Autodesk Inventor part; units mm, degrees
(part 5 of 8)
sketch "Skizze5" plane through (0, 0, 0) normal (0, 0, -1) x (-1, 0, 0)
  line L0 (4.6, 18.85) -> (4.6, 19.5)
  arc A0 (3.9, 18.15) -> (4.6, 18.85) centre (3.9, 18.85) ccw
  line L1 (-3.9, 18.15) -> (3.9, 18.15)
  arc A1 (-4.6, 18.85) -> (-3.9, 18.15) centre (-3.9, 18.85) ccw
  line L2 (-4.6, 19.5) -> (-4.6, 18.85)
  line L3 (-12.9, 19.5) -> (-4.6, 19.5)
  line L4 (-12.9, 14) -> (-12.9, 19.5)
  arc A2 (-14.1, 12.8) -> (-12.9, 14) centre (-14.1, 14) ccw
  line L5 (-15.5, 12.8) -> (-14.1, 12.8)
  line L6 (-15.5, -17) -> (-15.5, 12.8)
  line L7 (-13, -19.5) -> (-15.5, -17)
  line L8 (13, -19.5) -> (-13, -19.5)
  line L9 (15.5, -17) -> (13, -19.5)
  line L10 (15.5, 19.5) -> (15.5, -17)
  line L11 (4.6, 19.5) -> (15.5, 19.5)
  circle A3 centre (13.97, 2.98) radius 0.75
  circle A4 centre (13.97, 8.06) radius 0.75
  circle A5 centre (13.97, -4.64) radius 0.75
  circle A6 centre (-13.97, 8.06) radius 0.75
  circle A7 centre (-12.2, 14.85) radius 0.65
  circle A8 centre (-13.97, 0.44) radius 0.75
  circle A9 centre (-13.97, 5.52) radius 0.75
  circle A10 centre (-13.97, -2.1) radius 0.75
  line L12 (14.72, 9.85) -> (14.72, 11.35)
  line L13 (13.22, 9.85) -> (14.72, 9.85)
  line L14 (13.22, 11.35) -> (13.22, 9.85)
  line L15 (14.72, 11.35) -> (13.22, 11.35)
  circle A11 centre (13.97, -9.72) radius 0.75
  circle A12 centre (-13.97, -12.26) radius 0.75
  circle A13 centre (11.43, 8.06) radius 0.75
  circle A14 centre (-11.43, 8.06) radius 0.75
  line L16 (10.13, 5.52) -> (10.13, -12.26)
  arc A15 (12.73, 5.52) -> (10.13, 5.52) centre (11.43, 5.52) ccw
  line L17 (12.73, -12.26) -> (12.73, 5.52)
  arc A16 (10.13, -12.26) -> (12.73, -12.26) centre (11.43, -12.26) ccw
  spline S0 degree 3 poles (-6.6597, 8.2783) (-6.6601, 8.2679) (-6.6608, 8.2466) (-6.6655, 8.2142) (-6.6737, 8.1812) (-6.6829, 8.1533) (-6.6918, 8.1302) (-6.7001, 8.112) (-6.7094, 8.0929) (-6.7203, 8.0729) (-6.7319, 8.052) (-6.7451, 8.0303) (-6.7594, 8.0077) (-6.7697, 7.9925) (-6.7749, 7.9847) knots 0 0 0 0 0.09832 0.199417 0.305603 0.416162 0.474582 0.537006 0.603857 0.67409 0.749417 0.828253 0.912054 1 1 1 1
  line L18 (-6.7749, 7.9847) -> (-7.0828, 7.5344)
  line L19 (-7.0828, 7.5344) -> (-7.1545, 7.5842)
  line L20 (-7.1545, 7.5842) -> (-6.8765, 7.9907)
  spline S1 degree 3 poles (-6.8765, 7.9907) (-6.8942, 7.9885) (-6.9292, 7.9842) (-6.9643, 7.9835) (-6.9817, 7.9831) knots 0 0 0 0 0.507858 1 1 1 1
  spline S2 degree 3 poles (-6.9817, 7.9831) (-6.9922, 7.9833) (-7.0128, 7.9839) (-7.0431, 7.9881) (-7.0722, 7.9945) (-7.1, 8.0041) (-7.1267, 8.0161) (-7.1522, 8.0309) (-7.1764, 8.0483) (-7.1991, 8.0683) (-7.2198, 8.0902) (-7.2382, 8.1134) (-7.2535, 8.1381) (-7.2662, 8.1639) (-7.2758, 8.1911) (-7.2829, 8.2194) (-7.2872, 8.249) (-7.2877, 8.2691) (-7.2879, 8.2794) knots 0 0 0 0 0.066295 0.130131 0.192862 0.25436 0.31591 0.377338 0.440205 0.504175 0.568034 0.630228 0.690861 0.751422 0.811466 0.87275 0.935391 1 1 1 1
  spline S3 degree 3 poles (-7.2879, 8.2794) (-7.2875, 8.2933) (-7.2865, 8.3208) (-7.2787, 8.3609) (-7.2658, 8.3989) (-7.2478, 8.4345) (-7.2252, 8.4674) (-7.198, 8.497) (-7.1665, 8.5229) (-7.1312, 8.5452) (-7.0931, 8.5631) (-7.0532, 8.5763) (-7.0118, 8.5841) (-6.9838, 8.5851) (-6.9696, 8.5856) knots 0 0 0 0 0.085249 0.167327 0.248175 0.328829 0.409908 0.490584 0.572993 0.658265 0.744222 0.82906 0.913938 1 1 1 1
  spline S4 degree 3 poles (-6.9696, 8.5856) (-6.9558, 8.5851) (-6.9284, 8.5841) (-6.8882, 8.5765) (-6.8496, 8.5638) (-6.813, 8.5461) (-6.779, 8.524) (-6.7485, 8.4977) (-6.7221, 8.4672) (-6.6999, 8.4331) (-6.6821, 8.3965) (-6.6692, 8.3582) (-6.6612, 8.3187) (-6.6602, 8.2919) (-6.6597, 8.2783) knots 0 0 0 0 0.085532 0.169003 0.251943 0.335682 0.419409 0.501265 0.583703 0.668 0.751919 0.834598 0.916526 1 1 1 1
  line L21 (-3.0444, 5.02) -> (-3.0572, 5.02)
  line L22 (-3.0572, 5.02) -> (-3.4803, 6.02)
  line L23 (-3.4803, 6.02) -> (-3.3841, 6.02)
  line L24 (-3.3841, 6.02) -> (-3.0508, 5.2319)
  line L25 (-3.0508, 5.2319) -> (-2.7174, 6.02)
  line L26 (-2.7174, 6.02) -> (-2.6213, 6.02)
  line L27 (-2.6213, 6.02) -> (-3.0444, 5.02)
  spline S5 degree 3 poles (-3.7238, 5.7862) (-3.724, 5.7914) (-3.7242, 5.8018) (-3.7272, 5.817) (-3.7316, 5.8317) (-3.7378, 5.8459) (-3.746, 5.8595) (-3.7558, 5.8725) (-3.7675, 5.885) (-3.7809, 5.8966) (-3.7953, 5.9077) (-3.8111, 5.9171) (-3.8278, 5.9251) (-3.8454, 5.9318) (-3.864, 5.9368) (-3.8835, 5.9404) (-3.9039, 5.9426) (-3.9179, 5.9429) (-3.925, 5.9431) knots 0 0 0 0 0.055275 0.109966 0.163247 0.218076 0.273301 0.330909 0.390995 0.454176 0.518862 0.583311 0.648517 0.715031 0.782502 0.852323 0.924928 1 1 1 1
  spline S6 degree 3 poles (-3.925, 5.9431) (-3.9364, 5.9427) (-3.9586, 5.9419) (-3.9907, 5.9351) (-4.0205, 5.9243) (-4.0432, 5.9113) (-4.0601, 5.8985) (-4.0721, 5.8873) (-4.0839, 5.8749) (-4.0947, 5.8605) (-4.1056, 5.8451) (-4.1156, 5.8278) (-4.1253, 5.8092) (-4.1311, 5.796) (-4.1341, 5.7892) knots 0 0 0 0 0.122712 0.239685 0.351816 0.463766 0.520818 0.579448 0.640604 0.705298 0.773634 0.844669 0.920057 1 1 1 1
  line L28 (-4.1341, 5.7892) -> (-4.2238, 5.7892)
  spline S7 degree 3 poles (-4.2238, 5.7892) (-4.2214, 5.7993) (-4.2167, 5.819) (-4.2067, 5.8471) (-4.1959, 5.8737) (-4.183, 5.8983) (-4.1688, 5.9214) (-4.1526, 5.9424) (-4.1351, 5.962) (-4.1157, 5.9793) (-4.0954, 5.995) (-4.0739, 6.0084) (-4.0515, 6.0199) (-4.0282, 6.0294) (-4.0039, 6.0366) (-3.9788, 6.0418) (-3.9528, 6.0451) (-3.9351, 6.0455) (-3.9262, 6.0456) knots 0 0 0 0 0.072625 0.141977 0.208985 0.273957 0.336889 0.398745 0.460116 0.520825 0.580994 0.640152 0.698622 0.757271 0.816427 0.876254 0.937165 1 1 1 1
  spline S8 degree 3 poles (-3.9262, 6.0456) (-3.9131, 6.0452) (-3.8873, 6.0445) (-3.8494, 6.0373) (-3.8128, 6.0261) (-3.778, 6.0105) (-3.7456, 5.9913) (-3.7168, 5.9685) (-3.692, 5.9424) (-3.6712, 5.9136) (-3.6549, 5.8829) (-3.6428, 5.8512) (-3.6355, 5.8187) (-3.6346, 5.7968) (-3.6341, 5.7858) knots 0 0 0 0 0.090254 0.17854 0.266093 0.354631 0.441886 0.525747 0.608114 0.690197 0.770821 0.848326 0.924012 1 1 1 1
  spline S9 degree 3 poles (-3.6341, 5.7858) (-3.6344, 5.7753) (-3.6351, 5.7546) (-3.6406, 5.7244) (-3.6499, 5.6959) (-3.6628, 5.669) (-3.6795, 5.644) (-3.6996, 5.6206) (-3.7235, 5.5989) (-3.7416, 5.5865) (-3.7509, 5.5801) knots 0 0 0 0 0.128068 0.250608 0.37063 0.490072 0.610375 0.734313 0.863217 1 1 1 1
  spline S10 degree 3 poles (-3.7509, 5.5801) (-3.7403, 5.575) (-3.7192, 5.5648) (-3.6904, 5.5448) (-3.6644, 5.5218) (-3.6498, 5.5038) (-3.6425, 5.4948) knots 0 0 0 0 0.25388 0.503009 0.750291 1 1 1 1
  spline S11 degree 3 poles (-3.6425, 5.4948) (-3.6377, 5.4882) (-3.6282, 5.4751) (-3.6164, 5.4541) (-3.6057, 5.4329) (-3.5974, 5.4108) (-3.5909, 5.3882) (-3.5863, 5.365) (-3.5834, 5.3413) (-3.583, 5.3252) (-3.5828, 5.3171) knots 0 0 0 0 0.128136 0.254173 0.378112 0.501712 0.623986 0.747096 0.872875 1 1 1 1
  spline S12 degree 3 poles (-3.5828, 5.3171) (-3.5833, 5.3031) (-3.5844, 5.2751) (-3.5935, 5.2339) (-3.6077, 5.1935) (-3.6278, 5.1549) (-3.6523, 5.1188) (-3.6815, 5.0865) (-3.715, 5.0587) (-3.7524, 5.0355) (-3.7929, 5.017) (-3.8362, 5.0041) (-3.8817, 4.9957) (-3.9129, 4.9948) (-3.9288, 4.9944) knots 0 0 0 0 0.079648 0.158922 0.239619 0.322609 0.406035 0.487602 0.569685 0.653036 0.737436 0.822478 0.909748 1 1 1 1
  spline S13 degree 3 poles (-3.9288, 4.9944) (-3.9395, 4.9946) (-3.9605, 4.9951) (-3.9914, 4.9984) (-4.0209, 5.0045) (-4.0491, 5.0127) (-4.0759, 5.0231) (-4.1013, 5.0361) (-4.1254, 5.0513) (-4.1481, 5.069) (-4.1692, 5.0888) (-4.1883, 5.111) (-4.2056, 5.1353) (-4.2207, 5.1619) (-4.2343, 5.1905) (-4.2455, 5.2214) (-4.2554, 5.2544) (-4.26, 5.2774) (-4.2623, 5.2892) knots 0 0 0 0 0.065541 0.128963 0.190377 0.250092 0.308548 0.366398 0.424542 0.48317 0.542243 0.601739 0.662506 0.724856 0.789128 0.856346 0.926295 1 1 1 1
  line L29 (-4.2623, 5.2892) -> (-4.1726, 5.2892)
  spline S14 degree 3 poles (-4.1726, 5.2892) (-4.1702, 5.2815) (-4.1657, 5.2666) (-4.1579, 5.245) (-4.1491, 5.2252) (-4.1397, 5.2071) (-4.1297, 5.1905) (-4.1186, 5.1758) (-4.1071, 5.1623) (-4.0985, 5.1547) (-4.0942, 5.151) knots 0 0 0 0 0.14977 0.291316 0.425966 0.55216 0.671527 0.786122 0.895325 1 1 1 1
  spline S15 degree 3 poles (-4.0942, 5.151) (-4.0886, 5.1467) (-4.0775, 5.1381) (-4.0592, 5.1271) (-4.0401, 5.1175) (-4.0196, 5.1103) (-3.9981, 5.1041) (-3.9754, 5.1001) (-3.9517, 5.0973) (-3.9355, 5.097) (-3.9272, 5.0969) knots 0 0 0 0 0.118271 0.236178 0.355663 0.475904 0.600127 0.728608 0.861313 1 1 1 1
  spline S16 degree 3 poles (-3.9272, 5.0969) (-3.9178, 5.0971) (-3.8995, 5.0974) (-3.8728, 5.1006) (-3.8474, 5.1052) (-3.8236, 5.1123) (-3.801, 5.1211) (-3.7801, 5.1322) (-3.7604, 5.1451) (-3.7423, 5.1599) (-3.7261, 5.176) (-3.7117, 5.1928) (-3.6995, 5.2104) (-3.6897, 5.2287) (-3.682, 5.2476) (-3.6767, 5.2674) (-3.673, 5.2877) (-3.6727, 5.3015) (-3.6726, 5.3085) knots 0 0 0 0 0.076072 0.148752 0.218403 0.28576 0.350598 0.414964 0.478069 0.541761 0.60435 0.664075 0.721464 0.777587 0.832644 0.887844 0.94346 1 1 1 1
  spline S17 degree 3 poles (-3.6726, 5.3085) (-3.673, 5.3178) (-3.6739, 5.3364) (-3.6805, 5.3637) (-3.6915, 5.3901) (-3.7068, 5.415) (-3.7255, 5.438) (-3.7473, 5.4586) (-3.7725, 5.4756) (-3.7956, 5.4874) (-3.8161, 5.4954) (-3.8337, 5.5007) (-3.8533, 5.5052) (-3.8748, 5.5094) (-3.8983, 5.513) (-3.9239, 5.516) (-3.9514, 5.5184) (-3.9704, 5.5195) (-3.9803, 5.52) knots 0 0 0 0 0.066909 0.133485 0.201035 0.271234 0.34288 0.413836 0.485977 0.56023 0.599884 0.644055 0.691892 0.744688 0.801492 0.862858 0.929328 1 1 1 1
  line L30 (-3.9803, 5.52) -> (-3.9803, 5.6226)
  spline S18 degree 3 poles (-3.9803, 5.6226) (-3.9679, 5.6228) (-3.9437, 5.6232) (-3.9083, 5.6282) (-3.8744, 5.635) (-3.8429, 5.6456) (-3.8141, 5.6578) (-3.7891, 5.6721) (-3.7684, 5.6879) (-3.7518, 5.7056) (-3.7394, 5.7245) (-3.7303, 5.7443) (-3.7249, 5.765) (-3.7242, 5.7791) (-3.7238, 5.7862) knots 0 0 0 0 0.110166 0.215787 0.318027 0.417574 0.51165 0.596162 0.672935 0.74367 0.810677 0.874059 0.936696 1 1 1 1
  spline S19 degree 3 poles (-4.4738, 5.0072) (-4.4794, 5.0075) (-4.4903, 5.0081) (-4.506, 5.013) (-4.5204, 5.0206) (-4.5332, 5.0313) (-4.5436, 5.0441) (-4.5515, 5.0585) (-4.5562, 5.0741) (-4.5569, 5.085) (-4.5572, 5.0905) knots 0 0 0 0 0.127757 0.249414 0.372796 0.500111 0.62861 0.750643 0.873768 1 1 1 1
  spline S20 degree 3 poles (-4.5572, 5.0905) (-4.5569, 5.0962) (-4.5563, 5.1072) (-4.5515, 5.1229) (-4.5437, 5.1373) (-4.5331, 5.15) (-4.5204, 5.1606) (-4.506, 5.1683) (-4.4903, 5.1729) (-4.4794, 5.1735) (-4.4738, 5.1738) knots 0 0 0 0 0.129097 0.252046 0.373905 0.501038 0.628171 0.751376 0.872426 1 1 1 1
  spline S21 degree 3 poles (-4.4738, 5.1738) (-4.4683, 5.1735) (-4.4574, 5.1729) (-4.4416, 5.1684) (-4.4273, 5.1605) (-4.4146, 5.15) (-4.4041, 5.1372) (-4.3959, 5.123) (-4.3915, 5.1071) (-4.3908, 5.0961) (-4.3905, 5.0905) knots 0 0 0 0 0.127519 0.249986 0.371792 0.49887 0.625948 0.748492 0.870959 1 1 1 1
  spline S22 degree 3 poles (-4.3905, 5.0905) (-4.3909, 5.085) (-4.3915, 5.0742) (-4.3959, 5.0584) (-4.4041, 5.0442) (-4.4145, 5.0313) (-4.4273, 5.0207) (-4.4416, 5.0129) (-4.4573, 5.0081) (-4.4683, 5.0075) (-4.4738, 5.0072) knots 0 0 0 0 0.126178 0.248821 0.37154 0.499984 0.627244 0.749226 0.872298 1 1 1 1
  spline S23 degree 3 poles (-4.8649, 5.7862) (-4.865, 5.7914) (-4.8652, 5.8018) (-4.8682, 5.817) (-4.8727, 5.8317) (-4.8788, 5.8459) (-4.887, 5.8595) (-4.8968, 5.8725) (-4.9085, 5.885) (-4.922, 5.8966) (-4.9364, 5.9077) (-4.9521, 5.9171) (-4.9688, 5.9251) (-4.9865, 5.9318) (-5.0051, 5.9368) (-5.0246, 5.9404) (-5.045, 5.9426) (-5.0589, 5.9429) (-5.066, 5.9431) knots 0 0 0 0 0.055275 0.109966 0.163247 0.218076 0.273301 0.330909 0.390995 0.454176 0.518862 0.583311 0.648517 0.715031 0.782502 0.852323 0.924928 1 1 1 1
  spline S24 degree 3 poles (-5.066, 5.9431) (-5.0774, 5.9427) (-5.0996, 5.9419) (-5.1317, 5.9351) (-5.1615, 5.9243) (-5.1843, 5.9113) (-5.2011, 5.8985) (-5.2131, 5.8873) (-5.2249, 5.8749) (-5.2357, 5.8605) (-5.2467, 5.8451) (-5.2566, 5.8278) (-5.2663, 5.8092) (-5.2721, 5.796) (-5.2751, 5.7892) knots 0 0 0 0 0.122712 0.239685 0.351816 0.463766 0.520818 0.579448 0.640604 0.705298 0.773634 0.844669 0.920057 1 1 1 1
  line L31 (-5.2751, 5.7892) -> (-5.3649, 5.7892)
  spline S25 degree 3 poles (-5.3649, 5.7892) (-5.3624, 5.7993) (-5.3577, 5.819) (-5.3478, 5.8471) (-5.337, 5.8737) (-5.324, 5.8983) (-5.3099, 5.9214) (-5.2937, 5.9424) (-5.2761, 5.962) (-5.2568, 5.9793) (-5.2364, 5.995) (-5.2149, 6.0084) (-5.1925, 6.0199) (-5.1692, 6.0294) (-5.1449, 6.0366) (-5.1198, 6.0418) (-5.0938, 6.0451) (-5.0762, 6.0455) (-5.0672, 6.0456) knots 0 0 0 0 0.072625 0.141977 0.208985 0.273957 0.336889 0.398745 0.460116 0.520825 0.580994 0.640152 0.698622 0.757271 0.816427 0.876254 0.937165 1 1 1 1
  spline S26 degree 3 poles (-5.0672, 6.0456) (-5.0541, 6.0452) (-5.0283, 6.0445) (-4.9904, 6.0373) (-4.9538, 6.0261) (-4.919, 6.0105) (-4.8866, 5.9913) (-4.8579, 5.9685) (-4.833, 5.9424) (-4.8122, 5.9136) (-4.7959, 5.8829) (-4.7839, 5.8512) (-4.7766, 5.8187) (-4.7756, 5.7968) (-4.7751, 5.7858) knots 0 0 0 0 0.090254 0.17854 0.266093 0.354631 0.441886 0.525747 0.608114 0.690197 0.770821 0.848326 0.924012 1 1 1 1
  spline S27 degree 3 poles (-4.7751, 5.7858) (-4.7755, 5.7753) (-4.7761, 5.7546) (-4.7816, 5.7244) (-4.7909, 5.6959) (-4.8038, 5.669) (-4.8205, 5.644) (-4.8407, 5.6206) (-4.8645, 5.5989) (-4.8826, 5.5865) (-4.8919, 5.5801) knots 0 0 0 0 0.128068 0.250608 0.37063 0.490072 0.610375 0.734313 0.863217 1 1 1 1
  spline S28 degree 3 poles (-4.8919, 5.5801) (-4.8813, 5.575) (-4.8602, 5.5648) (-4.8315, 5.5448) (-4.8054, 5.5218) (-4.7908, 5.5038) (-4.7835, 5.4948) knots 0 0 0 0 0.25388 0.503009 0.750291 1 1 1 1
  spline S29 degree 3 poles (-4.7835, 5.4948) (-4.7787, 5.4882) (-4.7692, 5.4751) (-4.7574, 5.4541) (-4.7467, 5.4329) (-4.7384, 5.4108) (-4.7319, 5.3882) (-4.7273, 5.365) (-4.7245, 5.3413) (-4.7241, 5.3252) (-4.7238, 5.3171) knots 0 0 0 0 0.128136 0.254173 0.378112 0.501712 0.623986 0.747096 0.872875 1 1 1 1
  spline S30 degree 3 poles (-4.7238, 5.3171) (-4.7244, 5.3031) (-4.7254, 5.2751) (-4.7345, 5.2339) (-4.7487, 5.1935) (-4.7688, 5.1549) (-4.7934, 5.1188) (-4.8226, 5.0865) (-4.8561, 5.0587) (-4.8934, 5.0355) (-4.9339, 5.017) (-4.9772, 5.0041) (-5.0227, 4.9957) (-5.0539, 4.9948) (-5.0698, 4.9944) knots 0 0 0 0 0.079648 0.158922 0.239619 0.322609 0.406035 0.487602 0.569685 0.653036 0.737436 0.822478 0.909748 1 1 1 1
  spline S31 degree 3 poles (-5.0698, 4.9944) (-5.0805, 4.9946) (-5.1015, 4.9951) (-5.1325, 4.9984) (-5.162, 5.0045) (-5.1901, 5.0127) (-5.2169, 5.0231) (-5.2423, 5.0361) (-5.2665, 5.0513) (-5.2891, 5.069) (-5.3102, 5.0888) (-5.3293, 5.111) (-5.3466, 5.1353) (-5.3617, 5.1619) (-5.3754, 5.1905) (-5.3865, 5.2214) (-5.3964, 5.2544) (-5.401, 5.2774) (-5.4033, 5.2892) knots 0 0 0 0 0.065541 0.128963 0.190377 0.250092 0.308548 0.366398 0.424542 0.48317 0.542243 0.601739 0.662506 0.724856 0.789128 0.856346 0.926295 1 1 1 1
  line L32 (-5.4033, 5.2892) -> (-5.3136, 5.2892)
  spline S32 degree 3 poles (-5.3136, 5.2892) (-5.3113, 5.2815) (-5.3067, 5.2666) (-5.299, 5.245) (-5.2901, 5.2252) (-5.2807, 5.2071) (-5.2707, 5.1905) (-5.2596, 5.1758) (-5.2481, 5.1623) (-5.2395, 5.1547) (-5.2353, 5.151) knots 0 0 0 0 0.14977 0.291316 0.425966 0.55216 0.671527 0.786122 0.895325 1 1 1 1
  spline S33 degree 3 poles (-5.2353, 5.151) (-5.2297, 5.1467) (-5.2185, 5.1381) (-5.2003, 5.1271) (-5.1811, 5.1175) (-5.1606, 5.1103) (-5.1392, 5.1041) (-5.1165, 5.1001) (-5.0927, 5.0973) (-5.0765, 5.097) (-5.0682, 5.0969) knots 0 0 0 0 0.118271 0.236178 0.355663 0.475904 0.600127 0.728608 0.861313 1 1 1 1
  spline S34 degree 3 poles (-5.0682, 5.0969) (-5.0588, 5.0971) (-5.0405, 5.0974) (-5.0138, 5.1006) (-4.9884, 5.1052) (-4.9646, 5.1123) (-4.9421, 5.1211) (-4.9211, 5.1322) (-4.9014, 5.1451) (-4.8833, 5.1599) (-4.8671, 5.176) (-4.8528, 5.1928) (-4.8406, 5.2104) (-4.8307, 5.2287) (-4.823, 5.2476) (-4.8177, 5.2674) (-4.814, 5.2877) (-4.8137, 5.3015) (-4.8136, 5.3085) knots 0 0 0 0 0.076072 0.148752 0.218403 0.28576 0.350598 0.414964 0.478069 0.541761 0.60435 0.664075 0.721464 0.777587 0.832644 0.887844 0.94346 1 1 1 1
  spline S35 degree 3 poles (-4.8136, 5.3085) (-4.814, 5.3178) (-4.8149, 5.3364) (-4.8216, 5.3637) (-4.8325, 5.3901) (-4.8478, 5.415) (-4.8665, 5.438) (-4.8883, 5.4586) (-4.9135, 5.4756) (-4.9366, 5.4874) (-4.9571, 5.4954) (-4.9747, 5.5007) (-4.9943, 5.5052) (-5.0158, 5.5094) (-5.0394, 5.513) (-5.0649, 5.516) (-5.0924, 5.5184) (-5.1115, 5.5195) (-5.1213, 5.52) knots 0 0 0 0 0.066909 0.133485 0.201035 0.271234 0.34288 0.413836 0.485977 0.56023 0.599884 0.644055 0.691892 0.744688 0.801492 0.862858 0.929328 1 1 1 1
  line L33 (-5.1213, 5.52) -> (-5.1213, 5.6226)
  spline S36 degree 3 poles (-5.1213, 5.6226) (-5.1089, 5.6228) (-5.0847, 5.6232) (-5.0493, 5.6282) (-5.0154, 5.635) (-4.9839, 5.6456) (-4.9551, 5.6578) (-4.9302, 5.6721) (-4.9094, 5.6879) (-4.8929, 5.7056) (-4.8804, 5.7245) (-4.8713, 5.7443) (-4.8659, 5.765) (-4.8652, 5.7791) (-4.8649, 5.7862) knots 0 0 0 0 0.110166 0.215787 0.318027 0.417574 0.51165 0.596162 0.672935 0.74367 0.810677 0.874059 0.936696 1 1 1 1
  spline S37 degree 3 poles (-3.3905, 2.9796) (-3.3907, 2.9643) (-3.3911, 2.9345) (-3.3929, 2.8909) (-3.3966, 2.8498) (-3.4013, 2.811) (-3.4077, 2.7747) (-3.4156, 2.7408) (-3.4243, 2.7091) (-3.4351, 2.6798) (-3.447, 2.6527) (-3.4598, 2.6274) (-3.4736, 2.6036) (-3.4887, 2.5816) (-3.5047, 2.5612) (-3.522, 2.5428) (-3.5402, 2.5259) (-3.5595, 2.5109) (-3.5796, 2.4977) (-3.6002, 2.4859) (-3.6215, 2.4764) (-3.6432, 2.4683) (-3.6655, 2.462) (-3.6885, 2.4577) (-3.7119, 2.4547) (-3.7277, 2.4545) (-3.7357, 2.4544) knots 0 0 0 0 0.065063 0.126773 0.185516 0.240765 0.29298 0.34225 0.388919 0.432776 0.474628 0.514775 0.553606 0.591426 0.628028 0.663804 0.698984 0.733591 0.767628 0.801208 0.834264 0.866981 0.89972 0.932702 0.966176 1 1 1 1
  spline S38 degree 3 poles (-3.7357, 2.4544) (-3.7436, 2.4545) (-3.7591, 2.4548) (-3.7821, 2.4575) (-3.8045, 2.4618) (-3.8263, 2.468) (-3.8477, 2.4755) (-3.8683, 2.4852) (-3.8883, 2.4964) (-3.9079, 2.5092) (-3.9264, 2.5239) (-3.9442, 2.5401) (-3.9606, 2.5583) (-3.976, 2.5782) (-3.9905, 2.5995) (-4.0039, 2.6226) (-4.0163, 2.6474) (-4.0276, 2.6741) (-4.0377, 2.703) (-4.0465, 2.7345) (-4.0536, 2.7688) (-4.0595, 2.8057) (-4.0644, 2.8453) (-4.0677, 2.8877) (-4.0697, 2.9328) (-4.0699, 2.9637) (-4.07, 2.9796) knots 0 0 0 0 0.033787 0.066622 0.099285 0.131361 0.163585 0.196104 0.228902 0.262158 0.295991 0.330218 0.36506 0.400951 0.43762 0.475708 0.515381 0.556414 0.599765 0.646424 0.696431 0.749782 0.806573 0.867436 0.931887 1 1 1 1
  spline S39 degree 3 poles (-4.07, 2.9796) (-4.0699, 2.9956) (-4.0697, 3.0268) (-4.0677, 3.0721) (-4.0643, 3.1147) (-4.0597, 3.1544) (-4.0541, 3.1914) (-4.0466, 3.2255) (-4.0381, 3.2568) (-4.0282, 3.2855) (-4.0171, 3.312) (-4.005, 3.3366) (-3.9914, 3.3595) (-3.9771, 3.381) (-3.9616, 3.4007) (-3.9452, 3.4189) (-3.9273, 3.4351) (-3.9087, 3.45) (-3.8889, 3.4629) (-3.8688, 3.4744) (-3.848, 3.4841) (-3.8265, 3.4918) (-3.8046, 3.4982) (-3.7821, 3.5025) (-3.7591, 3.5052) (-3.7436, 3.5055) (-3.7357, 3.5056) knots 0 0 0 0 0.068595 0.133246 0.194313 0.251279 0.304513 0.354235 0.400481 0.443411 0.484015 0.523252 0.561042 0.5979 0.633518 0.668314 0.702496 0.736685 0.770293 0.803437 0.835913 0.86846 0.900847 0.933467 0.966258 1 1 1 1
  spline S40 degree 3 poles (-3.7357, 3.5056) (-3.7277, 3.5055) (-3.7119, 3.5052) (-3.6885, 3.5026) (-3.6657, 3.4981) (-3.6435, 3.4919) (-3.6217, 3.4841) (-3.6006, 3.4744) (-3.58, 3.463) (-3.5602, 3.4497) (-3.5409, 3.4349) (-3.5228, 3.4181) (-3.5058, 3.3995) (-3.4896, 3.3794) (-3.4747, 3.3573) (-3.4605, 3.3337) (-3.4479, 3.308) (-3.4356, 3.2808) (-3.4251, 3.2513) (-3.4156, 3.2197) (-3.4079, 3.1855) (-3.4015, 3.149) (-3.3966, 3.11) (-3.393, 3.0687) (-3.3911, 3.0249) (-3.3907, 2.995) (-3.3905, 2.9796) knots 0 0 0 0 0.033788 0.067194 0.099862 0.132567 0.165151 0.197913 0.231319 0.265083 0.299255 0.334399 0.369943 0.406284 0.444064 0.482998 0.523354 0.565537 0.609613 0.656391 0.705885 0.758325 0.813832 0.872795 0.934722 1 1 1 1
  spline S41 degree 3 poles (-2.7623, 0.7062) (-2.7624, 0.7114) (-2.7627, 0.7218) (-2.7656, 0.737) (-2.7701, 0.7517) (-2.7762, 0.7659) (-2.7844, 0.7795) (-2.7943, 0.7925) (-2.806, 0.805) (-2.8194, 0.8166) (-2.8338, 0.8277) (-2.8496, 0.8371) (-2.8663, 0.8451) (-2.8839, 0.8518) (-2.9025, 0.8568) (-2.922, 0.8604) (-2.9424, 0.8626) (-2.9563, 0.8629) (-2.9634, 0.8631) knots 0 0 0 0 0.055275 0.109966 0.163247 0.218076 0.273301 0.330909 0.390995 0.454176 0.518862 0.583311 0.648517 0.715031 0.782502 0.852323 0.924928 1 1 1 1
  spline S42 degree 3 poles (-2.9634, 0.8631) (-2.9748, 0.8627) (-2.9971, 0.8619) (-3.0291, 0.8551) (-3.0589, 0.8443) (-3.0817, 0.8313) (-3.0985, 0.8185) (-3.1106, 0.8073) (-3.1224, 0.7949) (-3.1332, 0.7805) (-3.1441, 0.7651) (-3.1541, 0.7478) (-3.1637, 0.7292) (-3.1696, 0.716) (-3.1726, 0.7092) knots 0 0 0 0 0.122712 0.239685 0.351816 0.463766 0.520818 0.579448 0.640604 0.705298 0.773634 0.844669 0.920057 1 1 1 1
  line L34 (-3.1726, 0.7092) -> (-3.2623, 0.7092)
  spline S43 degree 3 poles (-3.2623, 0.7092) (-3.2599, 0.7193) (-3.2551, 0.739) (-3.2452, 0.7671) (-3.2344, 0.7937) (-3.2214, 0.8183) (-3.2073, 0.8414) (-3.1911, 0.8624) (-3.1736, 0.882) (-3.1542, 0.8993) (-3.1339, 0.915) (-3.1123, 0.9284) (-3.09, 0.9399) (-3.0667, 0.9494) (-3.0423, 0.9566) (-3.0172, 0.9618) (-2.9912, 0.9651) (-2.9736, 0.9655) (-2.9646, 0.9656) knots 0 0 0 0 0.072625 0.141977 0.208985 0.273957 0.336889 0.398745 0.460116 0.520825 0.580994 0.640152 0.698622 0.757271 0.816427 0.876254 0.937165 1 1 1 1
  spline S44 degree 3 poles (-2.9646, 0.9656) (-2.9516, 0.9652) (-2.9258, 0.9645) (-2.8878, 0.9573) (-2.8512, 0.9461) (-2.8164, 0.9305) (-2.7841, 0.9113) (-2.7553, 0.8885) (-2.7305, 0.8624) (-2.7096, 0.8336) (-2.6933, 0.8029) (-2.6813, 0.7712) (-2.674, 0.7387) (-2.673, 0.7168) (-2.6726, 0.7058) knots 0 0 0 0 0.090254 0.17854 0.266093 0.354631 0.441886 0.525747 0.608114 0.690197 0.770821 0.848326 0.924012 1 1 1 1
  spline S45 degree 3 poles (-2.6726, 0.7058) (-2.6729, 0.6953) (-2.6735, 0.6746) (-2.6791, 0.6444) (-2.6884, 0.6159) (-2.7012, 0.589) (-2.7179, 0.564) (-2.7381, 0.5406) (-2.762, 0.5189) (-2.78, 0.5065) (-2.7894, 0.5001) knots 0 0 0 0 0.128068 0.250608 0.37063 0.490072 0.610375 0.734313 0.863217 1 1 1 1
  spline S46 degree 3 poles (-2.7894, 0.5001) (-2.7787, 0.495) (-2.7576, 0.4848) (-2.7289, 0.4648) (-2.7028, 0.4418) (-2.6883, 0.4238) (-2.681, 0.4148) knots 0 0 0 0 0.25388 0.503009 0.750291 1 1 1 1
  spline S47 degree 3 poles (-2.681, 0.4148) (-2.6762, 0.4082) (-2.6666, 0.3951) (-2.6548, 0.3741) (-2.6442, 0.3529) (-2.6358, 0.3308) (-2.6294, 0.3082) (-2.6248, 0.285) (-2.6219, 0.2613) (-2.6215, 0.2452) (-2.6213, 0.2371) knots 0 0 0 0 0.128136 0.254173 0.378112 0.501712 0.623986 0.747096 0.872875 1 1 1 1
  spline S48 degree 3 poles (-2.6213, 0.2371) (-2.6218, 0.2231) (-2.6228, 0.1951) (-2.632, 0.1539) (-2.6461, 0.1135) (-2.6663, 0.0749) (-2.6908, 0.0388) (-2.72, 0.0065) (-2.7535, -0.0213) (-2.7909, -0.0445) (-2.8314, -0.063) (-2.8747, -0.0759) (-2.9202, -0.0843) (-2.9514, -0.0852) (-2.9672, -0.0856) knots 0 0 0 0 0.079648 0.158922 0.239619 0.322609 0.406035 0.487602 0.569685 0.653036 0.737436 0.822478 0.909748 1 1 1 1
  spline S49 degree 3 poles (-2.9672, -0.0856) (-2.9779, -0.0854) (-2.999, -0.0849) (-3.0299, -0.0816) (-3.0594, -0.0755) (-3.0876, -0.0673) (-3.1144, -0.0569) (-3.1398, -0.0439) (-3.1639, -0.0287) (-3.1865, -0.011) (-3.2076, 0.0088) (-3.2267, 0.031) (-3.2441, 0.0553) (-3.2592, 0.0819) (-3.2728, 0.1105) (-3.284, 0.1414) (-3.2938, 0.1744) (-3.2984, 0.1974) (-3.3008, 0.2092) knots 0 0 0 0 0.065541 0.128963 0.190377 0.250092 0.308548 0.366398 0.424542 0.48317 0.542243 0.601739 0.662506 0.724856 0.789128 0.856346 0.926295 1 1 1 1
  line L35 (-3.3008, 0.2092) -> (-3.211, 0.2092)
  spline S50 degree 3 poles (-3.211, 0.2092) (-3.2087, 0.2015) (-3.2041, 0.1866) (-3.1964, 0.165) (-3.1876, 0.1452) (-3.1781, 0.1271) (-3.1682, 0.1105) (-3.1571, 0.0958) (-3.1456, 0.0823) (-3.1369, 0.0747) (-3.1327, 0.071) knots 0 0 0 0 0.14977 0.291316 0.425966 0.55216 0.671527 0.786122 0.895325 1 1 1 1
  spline S51 degree 3 poles (-3.1327, 0.071) (-3.1271, 0.0667) (-3.1159, 0.0581) (-3.0977, 0.0471) (-3.0785, 0.0375) (-3.058, 0.0303) (-3.0366, 0.0241) (-3.0139, 0.0201) (-2.9901, 0.0173) (-2.9739, 0.017) (-2.9656, 0.0169) knots 0 0 0 0 0.118271 0.236178 0.355663 0.475904 0.600127 0.728608 0.861313 1 1 1 1
  spline S52 degree 3 poles (-2.9656, 0.0169) (-2.9563, 0.0171) (-2.938, 0.0174) (-2.9113, 0.0206) (-2.8859, 0.0252) (-2.8621, 0.0323) (-2.8395, 0.0411) (-2.8185, 0.0522) (-2.7989, 0.0651) (-2.7808, 0.0799) (-2.7645, 0.096) (-2.7502, 0.1128) (-2.738, 0.1304) (-2.7282, 0.1487) (-2.7204, 0.1676) (-2.7151, 0.1874) (-2.7115, 0.2077) (-2.7112, 0.2215) (-2.711, 0.2285) knots 0 0 0 0 0.076072 0.148752 0.218403 0.28576 0.350598 0.414964 0.478069 0.541761 0.60435 0.664075 0.721464 0.777587 0.832644 0.887844 0.94346 1 1 1 1
  spline S53 degree 3 poles (-2.711, 0.2285) (-2.7115, 0.2378) (-2.7123, 0.2564) (-2.719, 0.2837) (-2.7299, 0.3101) (-2.7453, 0.335) (-2.764, 0.358) (-2.7858, 0.3786) (-2.8109, 0.3956) (-2.8341, 0.4074) (-2.8546, 0.4154) (-2.8721, 0.4207) (-2.8918, 0.4252) (-2.9133, 0.4294) (-2.9368, 0.433) (-2.9623, 0.436) (-2.9898, 0.4384) (-3.0089, 0.4395) (-3.0187, 0.44) knots 0 0 0 0 0.066909 0.133485 0.201035 0.271234 0.34288 0.413836 0.485977 0.56023 0.599884 0.644055 0.691892 0.744688 0.801492 0.862858 0.929328 1 1 1 1
  line L36 (-3.0187, 0.44) -> (-3.0187, 0.5426)
  spline S54 degree 3 poles (-3.0187, 0.5426) (-3.0063, 0.5428) (-2.9821, 0.5432) (-2.9467, 0.5482) (-2.9129, 0.555) (-2.8813, 0.5656) (-2.8526, 0.5778) (-2.8276, 0.5921) (-2.8068, 0.6079) (-2.7903, 0.6256) (-2.7779, 0.6445) (-2.7688, 0.6643) (-2.7634, 0.685) (-2.7627, 0.6991) (-2.7623, 0.7062) knots 0 0 0 0 0.110166 0.215787 0.318027 0.417574 0.51165 0.596162 0.672935 0.74367 0.810677 0.874059 0.936696 1 1 1 1
  spline S55 degree 3 poles (-3.4931, 0.6604) (-3.4933, 0.6672) (-3.4936, 0.6806) (-3.4968, 0.7003) (-3.5016, 0.7194) (-3.5084, 0.7377) (-3.5174, 0.7553) (-3.5284, 0.772) (-3.5411, 0.7882) (-3.5558, 0.8034) (-3.5719, 0.8173) (-3.5889, 0.8297) (-3.6069, 0.84) (-3.6259, 0.8484) (-3.6456, 0.855) (-3.6663, 0.8596) (-3.6878, 0.8625) (-3.7025, 0.8629) (-3.71, 0.8631) knots 0 0 0 0 0.061965 0.122122 0.180988 0.239933 0.299906 0.359989 0.421776 0.486576 0.551535 0.615018 0.677259 0.73973 0.80305 0.866495 0.931973 1 1 1 1
  spline S56 degree 3 poles (-3.71, 0.8631) (-3.7178, 0.8629) (-3.7332, 0.8625) (-3.7558, 0.8597) (-3.7773, 0.8548) (-3.7978, 0.8482) (-3.8174, 0.8398) (-3.8359, 0.8293) (-3.8533, 0.8168) (-3.8697, 0.8026) (-3.8848, 0.7868) (-3.8981, 0.7692) (-3.9097, 0.7501) (-3.9198, 0.7296) (-3.928, 0.7074) (-3.9343, 0.6837) (-3.9393, 0.6586) (-3.9409, 0.6412) (-3.9418, 0.6323) knots 0 0 0 0 0.064439 0.126547 0.186887 0.245878 0.304041 0.362191 0.420976 0.48066 0.5406 0.600689 0.661936 0.724443 0.789038 0.856314 0.926352 1 1 1 1
  line L37 (-3.9418, 0.6323) -> (-4.0315, 0.6323)
  spline S57 degree 3 poles (-4.0315, 0.6323) (-4.031, 0.6442) (-4.0298, 0.6676) (-4.0244, 0.7017) (-4.0167, 0.7343) (-4.0058, 0.7651) (-3.9923, 0.7944) (-3.9761, 0.8221) (-3.9569, 0.8481) (-3.9351, 0.8722) (-3.9115, 0.8942) (-3.886, 0.9133) (-3.8592, 0.9294) (-3.8311, 0.9428) (-3.8016, 0.9529) (-3.7708, 0.9604) (-3.7385, 0.9649) (-3.7166, 0.9654) (-3.7054, 0.9656) knots 0 0 0 0 0.068791 0.135103 0.198979 0.261904 0.323495 0.385195 0.446969 0.509765 0.572251 0.633405 0.693251 0.752583 0.812579 0.873275 0.93555 1 1 1 1
  spline S58 degree 3 poles (-3.7054, 0.9656) (-3.6945, 0.9654) (-3.6729, 0.9649) (-3.6415, 0.9605) (-3.6115, 0.9538) (-3.5832, 0.9442) (-3.5566, 0.9314) (-3.5316, 0.9161) (-3.5079, 0.8983) (-3.4866, 0.8774) (-3.467, 0.855) (-3.4501, 0.8312) (-3.4357, 0.8065) (-3.4236, 0.7809) (-3.4148, 0.7541) (-3.408, 0.7265) (-3.4042, 0.6977) (-3.4036, 0.6783) (-3.4033, 0.6684) knots 0 0 0 0 0.069475 0.136517 0.200789 0.26383 0.325735 0.387291 0.449509 0.512968 0.576275 0.63758 0.697903 0.757172 0.816599 0.876653 0.93729 1 1 1 1
  spline S59 degree 3 poles (-3.4033, 0.6684) (-3.4038, 0.6544) (-3.4048, 0.6268) (-3.413, 0.5863) (-3.4258, 0.5469) (-3.4412, 0.5153) (-3.4568, 0.4898) (-3.4708, 0.4688) (-3.4872, 0.4462) (-3.5063, 0.4221) (-3.5276, 0.3962) (-3.5513, 0.3686) (-3.5776, 0.3397) (-3.5961, 0.3199) (-3.6057, 0.3096) knots 0 0 0 0 0.098702 0.195672 0.292422 0.391343 0.444462 0.504229 0.570352 0.642546 0.722288 0.807921 0.90047 1 1 1 1
  line L38 (-3.6057, 0.3096) -> (-3.8559, 0.0426)
  line L39 (-3.8559, 0.0426) -> (-3.3905, 0.0426)
  line L40 (-3.3905, 0.0426) -> (-3.3905, -0.06)
  line L41 (-3.3905, -0.06) -> (-4.07, -0.06)
  line L42 (-4.07, -0.06) -> (-3.6822, 0.3539)
  spline S60 degree 3 poles (-3.6822, 0.3539) (-3.6727, 0.3637) (-3.6546, 0.3827) (-3.6289, 0.4103) (-3.6059, 0.4359) (-3.5853, 0.4595) (-3.5677, 0.4814) (-3.552, 0.5009) (-3.5394, 0.5188) (-3.5258, 0.5396) (-3.5126, 0.565) (-3.5012, 0.596) (-3.4943, 0.6279) (-3.4935, 0.6495) (-3.4931, 0.6604) knots 0 0 0 0 0.110803 0.212829 0.306101 0.390647 0.466924 0.534481 0.593587 0.644557 0.7362 0.825024 0.911986 1 1 1 1
  spline S61 degree 3 poles (-2.6597, -1.8817) (-2.6601, -1.8921) (-2.6608, -1.9134) (-2.6655, -1.9458) (-2.6737, -1.9788) (-2.6829, -2.0067) (-2.6918, -2.0298) (-2.7001, -2.048) (-2.7094, -2.0671) (-2.7203, -2.0871) (-2.7319, -2.108) (-2.7451, -2.1297) (-2.7594, -2.1523) (-2.7697, -2.1675) (-2.7749, -2.1753) knots 0 0 0 0 0.09832 0.199417 0.305603 0.416162 0.474582 0.537006 0.603857 0.67409 0.749417 0.828253 0.912054 1 1 1 1
  line L43 (-2.7749, -2.1753) -> (-3.0828, -2.6256)
  line L44 (-3.0828, -2.6256) -> (-3.1545, -2.5758)
  line L45 (-3.1545, -2.5758) -> (-2.8765, -2.1693)
  spline S62 degree 3 poles (-2.8765, -2.1693) (-2.8942, -2.1715) (-2.9292, -2.1758) (-2.9643, -2.1765) (-2.9817, -2.1769) knots 0 0 0 0 0.507858 1 1 1 1
  spline S63 degree 3 poles (-2.9817, -2.1769) (-2.9922, -2.1767) (-3.0128, -2.1761) (-3.0431, -2.1719) (-3.0722, -2.1655) (-3.1, -2.1559) (-3.1267, -2.1439) (-3.1522, -2.1291) (-3.1764, -2.1117) (-3.1991, -2.0917) (-3.2198, -2.0698) (-3.2382, -2.0466) (-3.2535, -2.0219) (-3.2662, -1.9961) (-3.2758, -1.9689) (-3.2829, -1.9406) (-3.2872, -1.911) (-3.2877, -1.8909) (-3.2879, -1.8806) knots 0 0 0 0 0.066295 0.130131 0.192862 0.25436 0.31591 0.377338 0.440205 0.504175 0.568034 0.630228 0.690861 0.751422 0.811466 0.87275 0.935391 1 1 1 1
  spline S64 degree 3 poles (-3.2879, -1.8806) (-3.2875, -1.8667) (-3.2865, -1.8392) (-3.2787, -1.7991) (-3.2658, -1.7611) (-3.2478, -1.7255) (-3.2252, -1.6926) (-3.198, -1.663) (-3.1665, -1.6371) (-3.1312, -1.6148) (-3.0931, -1.5969) (-3.0532, -1.5837) (-3.0118, -1.5759) (-2.9838, -1.5749) (-2.9696, -1.5744) knots 0 0 0 0 0.085249 0.167327 0.248175 0.328829 0.409908 0.490584 0.572993 0.658265 0.744222 0.82906 0.913938 1 1 1 1
  spline S65 degree 3 poles (-2.9696, -1.5744) (-2.9558, -1.5749) (-2.9284, -1.5759) (-2.8882, -1.5835) (-2.8496, -1.5962) (-2.813, -1.6139) (-2.779, -1.636) (-2.7485, -1.6623) (-2.7221, -1.6928) (-2.6999, -1.7269) (-2.6821, -1.7635) (-2.6692, -1.8018) (-2.6612, -1.8413) (-2.6602, -1.8681) (-2.6597, -1.8817) knots 0 0 0 0 0.085532 0.169003 0.251943 0.335682 0.419409 0.501265 0.583703 0.668 0.751919 0.834598 0.916526 1 1 1 1
  line L46 (-3.7623, -1.7026) -> (-3.9162, -1.7026)
  line L47 (-3.9162, -1.7026) -> (-3.8575, -1.6)
  line L48 (-3.8575, -1.6) -> (-3.6726, -1.6)
  line L49 (-3.6726, -1.6) -> (-3.6726, -2.6)
  line L50 (-3.6726, -2.6) -> (-3.7623, -2.6)
  line L51 (-3.7623, -2.6) -> (-3.7623, -1.7026)
  line L52 (-7.1854, -4.64) -> (-7.0828, -4.14)
  line L53 (-7.0828, -4.14) -> (-6.6726, -4.14)
  line L54 (-6.6726, -4.14) -> (-6.6726, -4.2426)
  line L55 (-6.6726, -4.2426) -> (-7.0127, -4.2426)
  line L56 (-7.0127, -4.2426) -> (-7.0666, -4.5056)
  spline S66 degree 3 poles (-7.0666, -4.5056) (-7.056, -4.5027) (-7.0355, -4.497) (-7.0052, -4.4907) (-6.9765, -4.4869) (-6.9578, -4.4864) (-6.9488, -4.4862) knots 0 0 0 0 0.275068 0.532901 0.773973 1 1 1 1
  spline S67 degree 3 poles (-6.9488, -4.4862) (-6.9376, -4.4864) (-6.9157, -4.4869) (-6.8836, -4.4914) (-6.8529, -4.4986) (-6.8237, -4.5087) (-6.7961, -4.5215) (-6.7701, -4.5375) (-6.7455, -4.5562) (-6.7227, -4.5778) (-6.7019, -4.6015) (-6.6837, -4.6269) (-6.6682, -4.6539) (-6.6558, -4.6827) (-6.6459, -4.713) (-6.6393, -4.7451) (-6.6348, -4.7786) (-6.6344, -4.8016) (-6.6341, -4.8133) knots 0 0 0 0 0.065808 0.129394 0.190894 0.251281 0.310815 0.370371 0.430768 0.492881 0.555104 0.616067 0.677256 0.73826 0.800762 0.864778 0.931045 1 1 1 1
  spline S68 degree 3 poles (-6.6341, -4.8133) (-6.6343, -4.8214) (-6.6347, -4.8376) (-6.6366, -4.8617) (-6.6403, -4.8852) (-6.6452, -4.9082) (-6.6517, -4.9307) (-6.6595, -4.9527) (-6.669, -4.9741) (-6.6795, -4.995) (-6.6913, -5.0151) (-6.7044, -5.0338) (-6.7182, -5.0516) (-6.733, -5.0681) (-6.7491, -5.0833) (-6.7662, -5.0973) (-6.7841, -5.1103) (-6.8031, -5.1218) (-6.8229, -5.1323) (-6.8436, -5.141) (-6.8649, -5.1487) (-6.887, -5.1549) (-6.9099, -5.1597) (-6.9336, -5.163) (-6.958, -5.1654) (-6.9745, -5.1656) (-6.9829, -5.1656) knots 0 0 0 0 0.044014 0.087434 0.130118 0.172554 0.214555 0.256298 0.298438 0.340849 0.382715 0.423924 0.464246 0.504074 0.543862 0.583567 0.623094 0.663229 0.703551 0.743938 0.784541 0.82575 0.867757 0.910745 0.954914 1 1 1 1
  spline S69 degree 3 poles (-6.9829, -5.1656) (-6.9928, -5.1654) (-7.0124, -5.1651) (-7.0411, -5.161) (-7.0688, -5.1552) (-7.0951, -5.1464) (-7.1204, -5.1355) (-7.1442, -5.1216) (-7.1672, -5.1059) (-7.1885, -5.0873) (-7.2083, -5.0671) (-7.226, -5.0451) (-7.2417, -5.0217) (-7.2553, -4.9969) (-7.2668, -4.9707) (-7.2759, -4.9429) (-7.2833, -4.9138) (-7.2864, -4.8938) (-7.2879, -4.8836) knots 0 0 0 0 0.065421 0.128708 0.190236 0.250724 0.310637 0.370766 0.431615 0.493523 0.555883 0.617342 0.678668 0.740711 0.802985 0.866803 0.932347 1 1 1 1
  line L57 (-7.2879, -4.8836) -> (-7.1982, -4.8836)
  spline S70 degree 3 poles (-7.1982, -4.8836) (-7.196, -4.8931) (-7.1918, -4.9115) (-7.1824, -4.9372) (-7.171, -4.9602) (-7.1575, -4.9806) (-7.1413, -4.9984) (-7.1229, -5.0143) (-7.1022, -5.0287) (-7.0793, -5.0406) (-7.055, -5.0508) (-7.0297, -5.0576) (-7.0039, -5.0624) (-6.9864, -5.0628) (-6.9777, -5.0631) knots 0 0 0 0 0.094687 0.181994 0.264377 0.34218 0.418618 0.496509 0.577369 0.661511 0.746733 0.831258 0.915206 1 1 1 1
  spline S71 degree 3 poles (-6.9777, -5.0631) (-6.9691, -5.0628) (-6.9522, -5.0624) (-6.9274, -5.0588) (-6.9035, -5.0534) (-6.8806, -5.0452) (-6.8585, -5.0352) (-6.8376, -5.0224) (-6.8173, -5.0077) (-6.7983, -4.9909) (-6.7809, -4.9723) (-6.7656, -4.9525) (-6.7528, -4.9313) (-6.742, -4.9092) (-6.7338, -4.8858) (-6.728, -4.8614) (-6.7246, -4.8358) (-6.7241, -4.8184) (-6.7238, -4.8095) knots 0 0 0 0 0.064207 0.126425 0.18768 0.248216 0.308305 0.369661 0.431699 0.495947 0.559758 0.622295 0.683911 0.745092 0.80674 0.869087 0.93329 1 1 1 1
  spline S72 degree 3 poles (-6.7238, -4.8095) (-6.724, -4.8014) (-6.7244, -4.7857) (-6.7274, -4.7628) (-6.7326, -4.741) (-6.7399, -4.7204) (-6.7491, -4.7009) (-6.7604, -4.6825) (-6.7739, -4.6655) (-6.7894, -4.6497) (-6.8063, -4.6352) (-6.825, -4.6228) (-6.8451, -4.6124) (-6.8663, -4.6034) (-6.8891, -4.597) (-6.9132, -4.5921) (-6.9387, -4.5893) (-6.9561, -4.5889) (-6.965, -4.5887) knots 0 0 0 0 0.065351 0.127916 0.18836 0.247216 0.30563 0.36377 0.422661 0.482687 0.5433 0.604118 0.664965 0.727413 0.791468 0.858055 0.927037 1 1 1 1
  spline S73 degree 3 poles (-6.965, -4.5887) (-6.9728, -4.5889) (-6.9888, -4.5892) (-7.0133, -4.5917) (-7.0391, -4.5958) (-7.0661, -4.6014) (-7.0943, -4.6087) (-7.1236, -4.6175) (-7.1542, -4.628) (-7.1748, -4.6359) (-7.1854, -4.64) knots 0 0 0 0 0.102203 0.211023 0.3251 0.446502 0.573788 0.708901 0.850358 1 1 1 1
  spline S74 degree 3 poles (-7.5315, -4.3738) (-7.5317, -4.3686) (-7.5319, -4.3582) (-7.5349, -4.343) (-7.5393, -4.3283) (-7.5455, -4.3141) (-7.5537, -4.3005) (-7.5635, -4.2875) (-7.5752, -4.275) (-7.5886, -4.2634) (-7.603, -4.2523) (-7.6188, -4.2429) (-7.6355, -4.2349) (-7.6531, -4.2282) (-7.6717, -4.2232) (-7.6912, -4.2196) (-7.7116, -4.2174) (-7.7256, -4.2171) (-7.7327, -4.2169) knots 0 0 0 0 0.055275 0.109966 0.163247 0.218076 0.273301 0.330909 0.390995 0.454176 0.518862 0.583311 0.648517 0.715031 0.782502 0.852323 0.924928 1 1 1 1
  spline S75 degree 3 poles (-7.7327, -4.2169) (-7.744, -4.2173) (-7.7663, -4.2181) (-7.7983, -4.2249) (-7.8282, -4.2357) (-7.8509, -4.2487) (-7.8678, -4.2615) (-7.8798, -4.2727) (-7.8916, -4.2851) (-7.9024, -4.2995) (-7.9133, -4.3149) (-7.9233, -4.3322) (-7.933, -4.3508) (-7.9388, -4.364) (-7.9418, -4.3708) knots 0 0 0 0 0.122712 0.239685 0.351816 0.463766 0.520818 0.579448 0.640604 0.705298 0.773634 0.844669 0.920057 1 1 1 1
  line L58 (-7.9418, -4.3708) -> (-8.0315, -4.3708)
  spline S76 degree 3 poles (-8.0315, -4.3708) (-8.0291, -4.3607) (-8.0244, -4.341) (-8.0144, -4.3129) (-8.0036, -4.2863) (-7.9907, -4.2617) (-7.9765, -4.2386) (-7.9603, -4.2176) (-7.9428, -4.198) (-7.9234, -4.1807) (-7.9031, -4.165) (-7.8815, -4.1516) (-7.8592, -4.1401) (-7.8359, -4.1306) (-7.8116, -4.1234) (-7.7865, -4.1182) (-7.7605, -4.1149) (-7.7428, -4.1145) (-7.7339, -4.1144) knots 0 0 0 0 0.072625 0.141977 0.208985 0.273957 0.336889 0.398745 0.460116 0.520825 0.580994 0.640152 0.698622 0.757271 0.816427 0.876254 0.937165 1 1 1 1
  spline S77 degree 3 poles (-7.7339, -4.1144) (-7.7208, -4.1148) (-7.695, -4.1155) (-7.6571, -4.1227) (-7.6205, -4.1339) (-7.5857, -4.1495) (-7.5533, -4.1687) (-7.5245, -4.1915) (-7.4997, -4.2176) (-7.4789, -4.2464) (-7.4626, -4.2771) (-7.4505, -4.3088) (-7.4432, -4.3413) (-7.4423, -4.3632) (-7.4418, -4.3742) knots 0 0 0 0 0.090254 0.17854 0.266093 0.354631 0.441886 0.525747 0.608114 0.690197 0.770821 0.848326 0.924012 1 1 1 1
  spline S78 degree 3 poles (-7.4418, -4.3742) (-7.4421, -4.3847) (-7.4428, -4.4054) (-7.4483, -4.4356) (-7.4576, -4.4641) (-7.4705, -4.491) (-7.4871, -4.516) (-7.5073, -4.5394) (-7.5312, -4.5611) (-7.5493, -4.5735) (-7.5586, -4.5799) knots 0 0 0 0 0.128068 0.250608 0.37063 0.490072 0.610375 0.734313 0.863217 1 1 1 1
  spline S79 degree 3 poles (-7.5586, -4.5799) (-7.5479, -4.585) (-7.5269, -4.5952) (-7.4981, -4.6152) (-7.4721, -4.6382) (-7.4575, -4.6562) (-7.4502, -4.6652) knots 0 0 0 0 0.25388 0.503009 0.750291 1 1 1 1
  spline S80 degree 3 poles (-7.4502, -4.6652) (-7.4454, -4.6718) (-7.4359, -4.6849) (-7.4241, -4.7059) (-7.4134, -4.7271) (-7.4051, -4.7492) (-7.3986, -4.7718) (-7.394, -4.795) (-7.3911, -4.8187) (-7.3907, -4.8348) (-7.3905, -4.8429) knots 0 0 0 0 0.128136 0.254173 0.378112 0.501712 0.623986 0.747096 0.872875 1 1 1 1
  spline S81 degree 3 poles (-7.3905, -4.8429) (-7.391, -4.8569) (-7.392, -4.8849) (-7.4012, -4.9261) (-7.4154, -4.9665) (-7.4355, -5.0051) (-7.46, -5.0412) (-7.4892, -5.0735) (-7.5227, -5.1013) (-7.5601, -5.1245) (-7.6006, -5.143) (-7.6439, -5.1559) (-7.6894, -5.1643) (-7.7206, -5.1652) (-7.7365, -5.1656) knots 0 0 0 0 0.079648 0.158922 0.239619 0.322609 0.406035 0.487602 0.569685 0.653036 0.737436 0.822478 0.909748 1 1 1 1
  spline S82 degree 3 poles (-7.7365, -5.1656) (-7.7472, -5.1654) (-7.7682, -5.1649) (-7.7991, -5.1616) (-7.8286, -5.1555) (-7.8568, -5.1473) (-7.8836, -5.1369) (-7.909, -5.1239) (-7.9331, -5.1087) (-7.9557, -5.091) (-7.9769, -5.0712) (-7.996, -5.049) (-8.0133, -5.0247) (-8.0284, -4.9981) (-8.042, -4.9695) (-8.0532, -4.9386) (-8.0631, -4.9056) (-8.0676, -4.8826) (-8.07, -4.8708) knots 0 0 0 0 0.065541 0.128963 0.190377 0.250092 0.308548 0.366398 0.424542 0.48317 0.542243 0.601739 0.662506 0.724856 0.789128 0.856346 0.926295 1 1 1 1
  line L59 (-8.07, -4.8708) -> (-7.9803, -4.8708)
  spline S83 degree 3 poles (-7.9803, -4.8708) (-7.9779, -4.8785) (-7.9734, -4.8934) (-7.9656, -4.915) (-7.9568, -4.9348) (-7.9473, -4.9529) (-7.9374, -4.9695) (-7.9263, -4.9842) (-7.9148, -4.9977) (-7.9062, -5.0053) (-7.9019, -5.009) knots 0 0 0 0 0.14977 0.291316 0.425966 0.55216 0.671527 0.786122 0.895325 1 1 1 1
  spline S84 degree 3 poles (-7.9019, -5.009) (-7.8963, -5.0133) (-7.8852, -5.0219) (-7.8669, -5.0329) (-7.8478, -5.0425) (-7.8273, -5.0497) (-7.8058, -5.0559) (-7.7831, -5.0599) (-7.7594, -5.0627) (-7.7432, -5.063) (-7.7349, -5.0631) knots 0 0 0 0 0.118271 0.236178 0.355663 0.475904 0.600127 0.728608 0.861313 1 1 1 1
  spline S85 degree 3 poles (-7.7349, -5.0631) (-7.7255, -5.0629) (-7.7072, -5.0626) (-7.6805, -5.0594) (-7.6551, -5.0548) (-7.6313, -5.0477) (-7.6087, -5.0389) (-7.5878, -5.0278) (-7.5681, -5.0149) (-7.55, -5.0001) (-7.5337, -4.984) (-7.5194, -4.9672) (-7.5072, -4.9496) (-7.4974, -4.9313) (-7.4897, -4.9124) (-7.4844, -4.8926) (-7.4807, -4.8723) (-7.4804, -4.8585) (-7.4803, -4.8515) knots 0 0 0 0 0.076072 0.148752 0.218403 0.28576 0.350598 0.414964 0.478069 0.541761 0.60435 0.664075 0.721464 0.777587 0.832644 0.887844 0.94346 1 1 1 1
  spline S86 degree 3 poles (-7.4803, -4.8515) (-7.4807, -4.8422) (-7.4816, -4.8236) (-7.4882, -4.7963) (-7.4992, -4.7699) (-7.5145, -4.745) (-7.5332, -4.722) (-7.555, -4.7014) (-7.5802, -4.6844) (-7.6033, -4.6726) (-7.6238, -4.6646) (-7.6414, -4.6593) (-7.661, -4.6548) (-7.6825, -4.6506) (-7.706, -4.647) (-7.7316, -4.644) (-7.7591, -4.6416) (-7.7781, -4.6405) (-7.7879, -4.64) knots 0 0 0 0 0.066909 0.133485 0.201035 0.271234 0.34288 0.413836 0.485977 0.56023 0.599884 0.644055 0.691892 0.744688 0.801492 0.862858 0.929328 1 1 1 1
  line L60 (-7.7879, -4.64) -> (-7.7879, -4.5374)
  spline S87 degree 3 poles (-7.7879, -4.5374) (-7.7756, -4.5372) (-7.7513, -4.5368) (-7.7159, -4.5318) (-7.6821, -4.525) (-7.6505, -4.5144) (-7.6218, -4.5022) (-7.5968, -4.4879) (-7.576, -4.4721) (-7.5595, -4.4544) (-7.5471, -4.4355) (-7.538, -4.4157) (-7.5326, -4.395) (-7.5319, -4.3809) (-7.5315, -4.3738) knots 0 0 0 0 0.110166 0.215787 0.318027 0.417574 0.51165 0.596162 0.672935 0.74367 0.810677 0.874059 0.936696 1 1 1 1
  spline S88 degree 3 poles (-2.9564, -4.1144) (-2.9437, -4.1148) (-2.9186, -4.1156) (-2.8818, -4.1224) (-2.8465, -4.1337) (-2.813, -4.1491) (-2.7817, -4.1681) (-2.7541, -4.1911) (-2.7297, -4.2168) (-2.7096, -4.2457) (-2.693, -4.2761) (-2.6814, -4.308) (-2.674, -4.3406) (-2.673, -4.3627) (-2.6726, -4.3738) knots 0 0 0 0 0.08941 0.176306 0.262626 0.349446 0.435498 0.518928 0.601355 0.684256 0.765807 0.844877 0.92228 1 1 1 1
  spline S89 degree 3 poles (-2.6726, -4.3738) (-2.673, -4.3846) (-2.6738, -4.4059) (-2.6806, -4.437) (-2.692, -4.4661) (-2.7075, -4.4935) (-2.7278, -4.5188) (-2.7526, -4.5423) (-2.7816, -4.5642) (-2.8034, -4.5765) (-2.8146, -4.5829) knots 0 0 0 0 0.121904 0.239413 0.35541 0.472091 0.592859 0.718703 0.854892 1 1 1 1
  spline S90 degree 3 poles (-2.8146, -4.5829) (-2.8064, -4.5872) (-2.7904, -4.5955) (-2.7677, -4.6089) (-2.7469, -4.623) (-2.7275, -4.6372) (-2.7099, -4.652) (-2.6941, -4.6674) (-2.6799, -4.6831) (-2.6675, -4.6994) (-2.6566, -4.7161) (-2.6471, -4.7334) (-2.6391, -4.7512) (-2.6327, -4.7697) (-2.6274, -4.7886) (-2.6238, -4.8082) (-2.6218, -4.8283) (-2.6215, -4.8419) (-2.6213, -4.8487) knots 0 0 0 0 0.079525 0.1551 0.22722 0.295911 0.362056 0.42552 0.485813 0.544495 0.60146 0.657841 0.713974 0.769468 0.82613 0.882885 0.940701 1 1 1 1
  spline S91 degree 3 poles (-2.6213, -4.8487) (-2.6215, -4.8584) (-2.6219, -4.8774) (-2.6257, -4.9055) (-2.6314, -4.9329) (-2.6397, -4.9594) (-2.6505, -4.9849) (-2.6638, -5.0095) (-2.6788, -5.0336) (-2.6909, -5.0484) (-2.697, -5.0559) knots 0 0 0 0 0.128158 0.253673 0.377325 0.499385 0.622918 0.745839 0.871395 1 1 1 1
  spline S92 degree 3 poles (-2.697, -5.0559) (-2.705, -5.0646) (-2.7208, -5.082) (-2.7478, -5.1045) (-2.7776, -5.1235) (-2.8098, -5.1389) (-2.8445, -5.151) (-2.8816, -5.1596) (-2.9212, -5.1646) (-2.9485, -5.1653) (-2.9624, -5.1656) knots 0 0 0 0 0.119283 0.237093 0.354796 0.474576 0.59746 0.724926 0.858883 1 1 1 1
  spline S93 degree 3 poles (-2.9624, -5.1656) (-2.9759, -5.1653) (-3.002, -5.1647) (-3.04, -5.1603) (-3.0755, -5.1527) (-3.1086, -5.1423) (-3.1391, -5.1288) (-3.167, -5.1119) (-3.1926, -5.0924) (-3.2151, -5.0697) (-3.2351, -5.0454) (-3.2527, -5.0203) (-3.2673, -4.9945) (-3.2797, -4.9683) (-3.2892, -4.9413) (-3.2958, -4.9137) (-3.2999, -4.8855) (-3.3005, -4.8665) (-3.3008, -4.8569) knots 0 0 0 0 0.078556 0.152863 0.22356 0.290375 0.355403 0.418291 0.480389 0.543073 0.604924 0.664398 0.721943 0.778375 0.83383 0.888861 0.944089 1 1 1 1
  spline S94 degree 3 poles (-3.3008, -4.8569) (-3.3006, -4.8499) (-3.3003, -4.8361) (-3.298, -4.8156) (-3.2944, -4.7956) (-3.2895, -4.7762) (-3.2828, -4.7573) (-3.2747, -4.739) (-3.2653, -4.7212) (-3.2544, -4.7037) (-3.2418, -4.687) (-3.2274, -4.6706) (-3.2111, -4.6548) (-3.1931, -4.6394) (-3.1734, -4.6243) (-3.1517, -4.61) (-3.1284, -4.5958) (-3.1119, -4.5873) (-3.1035, -4.5829) knots 0 0 0 0 0.058854 0.116315 0.172675 0.22878 0.28458 0.340257 0.39663 0.453507 0.512318 0.572648 0.636022 0.702363 0.771483 0.844184 0.92007 1 1 1 1
  spline S95 degree 3 poles (-3.1035, -4.5829) (-3.1151, -4.5766) (-3.1375, -4.5643) (-3.1672, -4.5418) (-3.1928, -4.5175) (-3.2134, -4.4907) (-3.2297, -4.4624) (-3.2408, -4.4328) (-3.2484, -4.4023) (-3.2491, -4.3814) (-3.2495, -4.371) knots 0 0 0 0 0.14586 0.282426 0.41085 0.535029 0.654701 0.770133 0.884556 1 1 1 1
  spline S96 degree 3 poles (-3.2495, -4.371) (-3.249, -4.3603) (-3.2481, -4.3389) (-3.2405, -4.307) (-3.2281, -4.2757) (-3.2113, -4.2451) (-3.1903, -4.2162) (-3.1651, -4.1904) (-3.1364, -4.1677) (-3.1042, -4.1487) (-3.0696, -4.1332) (-3.033, -4.1225) (-2.9952, -4.1156) (-2.9695, -4.1148) (-2.9564, -4.1144) knots 0 0 0 0 0.074058 0.14887 0.226668 0.307735 0.391157 0.473929 0.557928 0.644989 0.733364 0.821092 0.909287 1 1 1 1
  line L61 (-3.7623, -4.2426) -> (-3.9162, -4.2426)
  line L62 (-3.9162, -4.2426) -> (-3.8575, -4.14)
  line L63 (-3.8575, -4.14) -> (-3.6726, -4.14)
  line L64 (-3.6726, -4.14) -> (-3.6726, -5.14)
  line L65 (-3.6726, -5.14) -> (-3.7623, -5.14)
  line L66 (-3.7623, -5.14) -> (-3.7623, -4.2426)
  spline S97 degree 3 poles (-3.2495, -7.4012) (-3.2491, -7.3909) (-3.2485, -7.3698) (-3.2436, -7.338) (-3.2359, -7.3054) (-3.2273, -7.2778) (-3.2181, -7.2551) (-3.2105, -7.2368) (-3.201, -7.2181) (-3.1909, -7.1981) (-3.1793, -7.1775) (-3.1666, -7.1558) (-3.1526, -7.1335) (-3.1427, -7.1184) (-3.1377, -7.1107) knots 0 0 0 0 0.097818 0.199726 0.305276 0.415811 0.474472 0.537274 0.603657 0.674299 0.749834 0.828598 0.912378 1 1 1 1
  line L67 (-3.1377, -7.1107) -> (-2.8392, -6.6544)
  line L68 (-2.8392, -6.6544) -> (-2.7701, -6.7086)
  line L69 (-2.7701, -6.7086) -> (-3.0343, -7.1127)
  spline S98 degree 3 poles (-3.0343, -7.1127) (-3.0168, -7.1099) (-2.9824, -7.1044) (-2.9477, -7.1035) (-2.9308, -7.1031) knots 0 0 0 0 0.512659 1 1 1 1
  spline S99 degree 3 poles (-2.9308, -7.1031) (-2.9206, -7.1034) (-2.9006, -7.1039) (-2.8712, -7.108) (-2.843, -7.1145) (-2.816, -7.1241) (-2.7903, -7.1362) (-2.7655, -7.1508) (-2.7422, -7.1685) (-2.7201, -7.1883) (-2.7, -7.2102) (-2.6823, -7.2334) (-2.6673, -7.258) (-2.6552, -7.2839) (-2.6458, -7.311) (-2.639, -7.3394) (-2.6349, -7.369) (-2.6344, -7.3891) (-2.6341, -7.3994) knots 0 0 0 0 0.065231 0.128405 0.190067 0.250943 0.311546 0.372863 0.435024 0.499072 0.563091 0.62551 0.68668 0.747283 0.808563 0.870742 0.934341 1 1 1 1
  spline S100 degree 3 poles (-2.6341, -7.3994) (-2.6345, -7.4133) (-2.6353, -7.4409) (-2.6433, -7.481) (-2.6557, -7.5192) (-2.6734, -7.5549) (-2.6954, -7.588) (-2.7222, -7.6174) (-2.7529, -7.6436) (-2.7876, -7.6655) (-2.825, -7.6834) (-2.8642, -7.6962) (-2.905, -7.7041) (-2.9326, -7.7051) (-2.9466, -7.7056) knots 0 0 0 0 0.085948 0.169125 0.250399 0.33229 0.413364 0.494172 0.576022 0.660757 0.745783 0.830044 0.914028 1 1 1 1
  spline S101 degree 3 poles (-2.9466, -7.7056) (-2.9601, -7.7052) (-2.9867, -7.7043) (-3.0259, -7.6966) (-3.0636, -7.6841) (-3.0995, -7.6669) (-3.1327, -7.6452) (-3.1624, -7.6191) (-3.1885, -7.589) (-3.2102, -7.5551) (-3.2274, -7.5187) (-3.2404, -7.4807) (-3.2479, -7.4413) (-3.249, -7.4146) (-3.2495, -7.4012) knots 0 0 0 0 0.084335 0.167052 0.249566 0.33274 0.415915 0.497828 0.580373 0.6646 0.749467 0.83251 0.915639 1 1 1 1
  spline S102 degree 3 poles (-3.4931, -6.9596) (-3.4933, -6.9528) (-3.4936, -6.9394) (-3.4968, -6.9197) (-3.5016, -6.9006) (-3.5084, -6.8823) (-3.5174, -6.8647) (-3.5284, -6.848) (-3.5411, -6.8318) (-3.5558, -6.8166) (-3.5719, -6.8027) (-3.5889, -6.7903) (-3.6069, -6.78) (-3.6259, -6.7716) (-3.6456, -6.765) (-3.6663, -6.7604) (-3.6878, -6.7575) (-3.7025, -6.7571) (-3.71, -6.7569) knots 0 0 0 0 0.061965 0.122122 0.180988 0.239933 0.299906 0.359989 0.421776 0.486576 0.551535 0.615018 0.677259 0.73973 0.80305 0.866495 0.931973 1 1 1 1
  spline S103 degree 3 poles (-3.71, -6.7569) (-3.7178, -6.7571) (-3.7332, -6.7575) (-3.7558, -6.7603) (-3.7773, -6.7652) (-3.7978, -6.7718) (-3.8174, -6.7802) (-3.8359, -6.7907) (-3.8533, -6.8032) (-3.8697, -6.8174) (-3.8848, -6.8332) (-3.8981, -6.8508) (-3.9097, -6.8699) (-3.9198, -6.8904) (-3.928, -6.9126) (-3.9343, -6.9363) (-3.9393, -6.9614) (-3.9409, -6.9788) (-3.9418, -6.9877) knots 0 0 0 0 0.064439 0.126547 0.186887 0.245878 0.304041 0.362191 0.420976 0.48066 0.5406 0.600689 0.661936 0.724443 0.789038 0.856314 0.926352 1 1 1 1
  line L70 (-3.9418, -6.9877) -> (-4.0315, -6.9877)
  spline S104 degree 3 poles (-4.0315, -6.9877) (-4.031, -6.9758) (-4.0298, -6.9524) (-4.0244, -6.9183) (-4.0167, -6.8857) (-4.0058, -6.8549) (-3.9923, -6.8256) (-3.9761, -6.7979) (-3.9569, -6.7719) (-3.9351, -6.7478) (-3.9115, -6.7258) (-3.886, -6.7067) (-3.8592, -6.6906) (-3.8311, -6.6772) (-3.8016, -6.6671) (-3.7708, -6.6596) (-3.7385, -6.6551) (-3.7166, -6.6546) (-3.7054, -6.6544) knots 0 0 0 0 0.068791 0.135103 0.198979 0.261904 0.323495 0.385195 0.446969 0.509765 0.572251 0.633405 0.693251 0.752583 0.812579 0.873275 0.93555 1 1 1 1